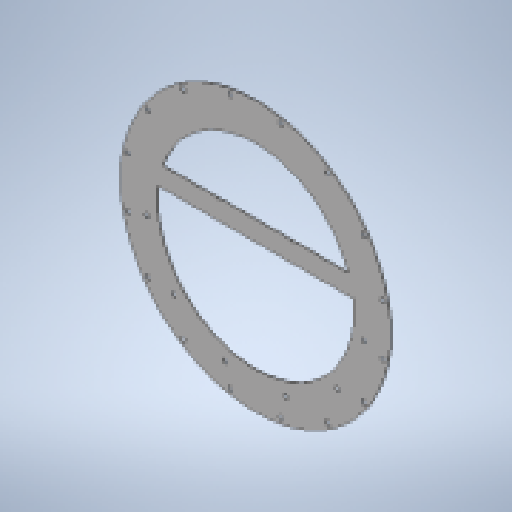
# Autodesk Inventor part: DMF 2.1 01 45 Gear ring 5_CPY
Saved by Autodesk Inventor 2026.2 (Build 302298000, 298)
## iProperties
Created: 2024-04-30
Part Number: DMF 2.1 01 45 Gear ring 5_CPY
Material: Generic
Document SubType Name: Sheet Metal
Designer: admin
Stock Number: Барабан_Сектор_Усилителя
Density: 1 g/cm^3
Flat Pattern Width: 55 cm
Flat Pattern Length: 55 cm
Flat Pattern Area: 3025 cm^2
Sheet Metal Rule: Default
Sheet Metal Width: 550,000 mm
Sheet Metal Length: 550,000 mm
Sheet Metal Area: 302500,000 mm^2
Appearance: Default
Author: pokla
Autodesk Inventor part; units mm, degrees
ref_plane "YZ Plane" through (0, 0, 0) normal (1, 0, 0) x (0, 1, 0)
ref_plane "XZ Plane" through (0, 0, 0) normal (0, 1, 0) x (-1, 0, 0)
ref_plane "XY Plane" through (0, 0, 0) normal (0, 0, 1) x (1, 0, 0)
sketch "Sketch1" plane through (0, 0, 0) normal (0, 0, 1) x (1, 0, 0)
  circle A0 centre (0, 0) radius 200
  circle A1 centre (0, 0) radius 275
  circle A2 centre (0, 0) radius 265 construction
  line L0 (-158.7713, -275) -> (-317.5426, 0) construction
  line L1 (-317.5426, 0) -> (-158.7713, 275) construction
  line L2 (-158.7713, 275) -> (158.7713, 275) construction
  line L3 (158.7713, 275) -> (317.5426, 0) construction
  line L4 (317.5426, 0) -> (158.7713, -275) construction
  line L5 (158.7713, -275) -> (-158.7713, -275) construction
  arc A3 (-33.4427, 262.8813) -> (-69.7033, 255.6686) centre (0, 0) ccw construction
  arc A4 (-34.0611, 267.7421) -> (-70.9921, 260.3961) centre (0, 0) ccw construction
  arc A5 (-32.8244, 258.0205) -> (-68.4144, 250.9412) centre (0, 0) ccw construction
  arc A6 (-32.8244, 258.0205) -> (-34.0611, 267.7421) centre (-33.4427, 262.8813) ccw construction
  arc A7 (-70.9921, 260.3961) -> (-68.4144, 250.9412) centre (-69.7033, 255.6686) ccw construction
  line L6 (-33.4427, 262.8813) -> (0, 0) construction
  line L7 (-69.7033, 255.6686) -> (0, 0) construction
  line L8 (0, 0) -> (0, 200) construction
  line L9 (-51.6989, 259.9081) -> (0, 0) construction
  circle A8 centre (-51.6989, 259.9081) radius 4.9
  circle A9 centre (-147.2261, 220.3394) radius 4.9
  circle A10 centre (-220.3394, 147.2261) radius 4.9
  circle A11 centre (-259.9081, 51.6989) radius 4.9
  circle A12 centre (-259.9081, -51.6989) radius 4.9
  circle A13 centre (-220.3394, -147.2261) radius 4.9
  circle A14 centre (-147.2261, -220.3394) radius 4.9
  circle A15 centre (-51.6989, -259.9081) radius 4.9
  circle A16 centre (51.6989, -259.9081) radius 4.9
  circle A17 centre (147.2261, -220.3394) radius 4.9
  circle A18 centre (220.3394, -147.2261) radius 4.9
  circle A19 centre (259.9081, -51.6989) radius 4.9
  circle A20 centre (259.9081, 51.6989) radius 4.9
  circle A21 centre (220.3394, 147.2261) radius 4.9
  circle A22 centre (147.2261, 220.3394) radius 4.9
  circle A23 centre (51.6989, 259.9081) radius 4.9
  circle A24 centre (-221.5817, -39.0708) radius 4.9
  circle A25 centre (0, 0) radius 225 construction
  line L10 (0, 0) -> (-275, 0) construction
  line L11 (-221.5817, -39.0708) -> (0, 0) construction
  circle A26 centre (-167.2076, -150.5544) radius 4.9
  circle A27 centre (-62.0184, -216.2839) radius 4.9
  circle A28 centre (62.0184, -216.2839) radius 4.9
  circle A29 centre (167.2076, -150.5544) radius 4.9
  circle A30 centre (221.5817, -39.0708) radius 4.9
  line L12 (-189.1428, 65) -> (198.4313, 65)
  line L13 (198.4313, 65) -> (198.4313, 25)
  line L14 (198.4313, 25) -> (-189.1428, 25)
  line L15 (-189.1428, 25) -> (-189.1428, 65)
  line L16 (-189.1428, 25) -> (-198.4313, 25)
  line L17 (72.5, 65) -> (72.5, 63)
  line L18 (72.5, 63) -> (75.5, 63)
  line L19 (75.5, 63) -> (75.5, 65)
  line L20 (-75.5, 65) -> (-75.5, 63)
  line L21 (-75.5, 63) -> (-72.5, 63)
  line L22 (-72.5, 63) -> (-72.5, 65)
  point P0 (0, -275)
  point P1 (238.157, 137.5)
  point P2 (-238.157, 137.5)
  point P3 (-189.1428, 45)
  point P4 (-198.9975, -20)
  point P5 (189.1428, 65)
  point P6 (74, 63)
  point P7 (-74, 63)
  dimension "d39" = 530
  dimension "d84" = 450
  dimension "d31" = 550
  dimension "d32" = 400
  dimension "d57" = 8
  dimension "d58" = 11.25
  dimension "d82" = 360
  dimension "d89" = 10
  dimension "d92" = 160
  dimension "d94" = 9.8
  dimension "d95" = 40
  dimension "d96" = 25
  dimension "d97" = 2
  dimension "d98" = 3
  dimension "d99" = 148
  measures "d31" diameter of A1
  measures "d32" diameter of A0
  measures "d57" angle of L7 L6
  measures "d58" angle of L8 L9
  measures "d89" angle of L11 L10
  measures "d94" diameter of A8
  measures "d95" distance of L14.end L12.start
  measures "d96" distance from line of point (0, 0) L14
  measures "d97" distance of L17.start L17.end
  measures "d98" distance of L17.end L18.end
  measures "d99" distance of point (74, 63) point (-74, 63)
extrude "Plate4" add sketch "Sketch1" along normal blind 2 contours L14 L15 L12 L20 L21 L22 L17 L18 L19 A0 | A0 L12 L13 | A0 L15 L16 | A1
sketch "Sketch5" plane through (0, 0, 2) normal (0, 0, 1) x (1, 0, 0)
  line L0 (-1.6, -169) -> (1.6, -169)
  line L1 (1.6, -169) -> (1.6, -209)
  line L2 (1.6, -209) -> (-1.6, -209)
  line L3 (-1.6, -209) -> (-1.6, -169)
  line L4 (-207, -40) -> (-167, -40)
  line L5 (-167, -40) -> (-167, -43.2)
  line L6 (-167, -43.2) -> (-207, -43.2)
  line L7 (-207, -43.2) -> (-207, -40)
  line L8 (0, 0) -> (0, -169)
  line L9 (167, -40) -> (207, -40)
  line L10 (207, -40) -> (207, -43.2)
  line L11 (207, -43.2) -> (167, -43.2)
  line L12 (167, -43.2) -> (167, -40)
  dimension "d74" = 3.2
  dimension "d75" = 40
  dimension "d76" = 40
  dimension "d77" = 40
  dimension "d78" = 167
  dimension "d79" = 169
  constraints: 26 end point, 6 parallel, 3 equal length, 3 horizontal, 3 perpendicular, 1 collinear, 1 midpoint, 1 vertical, 1 other
  measures "d74" distance of L0.start L0.end
  measures "d75" distance of L0.end L1.end
  measures "d76" distance of L4.start L4.end
  measures "d77" distance from line of L8.start L4
  measures "d78" distance between parallel lines of L8 L5
  measures "d79" distance from line of L0 L8.start
feature "Mark1" [suppressed]
equation "\"d63\" = Thickness"
equation "\"BendRadius\" = Thickness"
equation "\"BendReliefWidth\" = Thickness"
equation "\"BendReliefDepth\" = 0.5 * Thickness"
equation "\"CornerReliefSize\" = 4 * Thickness"
equation "\"MinimumRemnant\" = 2 * Thickness"
equation "\"TransitionRadius\" = BendRadius"
equation "\"JacobiRadiusSize\" = BendRadius"
equation "\"GapSize\" = Thickness"
equation "\"Thickness\" = 2"
body "Solid3"
